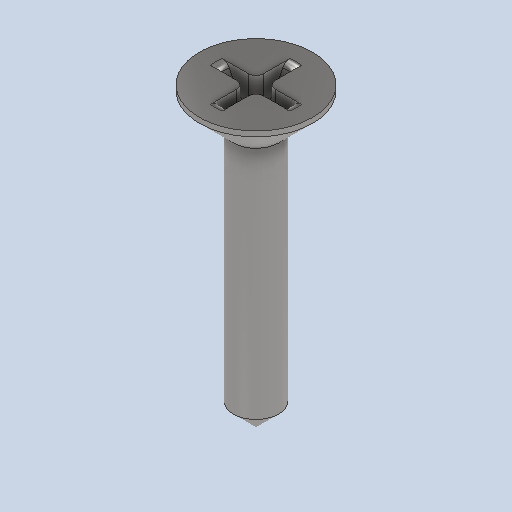
# Autodesk Inventor part: screw EE
Saved by Autodesk Inventor 2022 (Build 260153000, 153)
## iProperties
Created: 2021-06-28
Part Number: screw EE
Material: Iron, Malleable
Document SubType Name: Modeling
Designer: HP
Density: 7.15 g/cm^3
Appearance: Semi-Polished
Author: HP
Autodesk Inventor part; units mm, degrees
ref_plane "YZ Plane" through (0, 0, 0) normal (1, 0, 0) x (0, 1, 0)
ref_plane "XZ Plane" through (0, 0, 0) normal (0, 1, 0) x (-1, 0, 0)
ref_plane "XY Plane" through (0, 0, 0) normal (0, 0, 1) x (1, 0, 0)
sketch "Sketch1" plane through (0, 0, 0) normal (0, 0, 1) x (1, 0, 0)
  line L0 (0, -2.5) -> (0, -19)
  line L1 (0, -19) -> (1.4515, -17.5485)
  line L2 (1.4515, -17.5485) -> (1.4515, -2.5)
  line L3 (1.4515, -2.5) -> (3.625, -0.3265)
  line L4 (3.625, -0.3265) -> (3.625, 0)
  line L5 (3.625, 0) -> (2.25, 0)
  line L6 (0.7598, -2.0613) -> (0, -2.5)
  line L7 (0.7598, -2.0613) -> (1.5664, -1.466)
  line L8 (1.5664, -1.466) -> (2.25, 0)
  point P0 (0, 0)
  dimension "d0" = 3.625
  dimension "d1" = 2.25
  dimension "d2" = 19
  dimension "d3" = 60
  dimension "d4" = 45
  dimension "d5" = 2.5
  dimension "d6" = 2.5
  dimension "d7" = 25
  constraints: 18 end point, 3 parallel, 2 point on line, 1 perpendicular, 1 vertical
  measures "d0" distance from line of L0 L4.end
  measures "d1" distance from line of L0 L5.end
  measures "d2" distance from line of L0.end L5
  measures "d3" angle of L0 L6
  measures "d4" angle of L0 L3
  measures "d5" distance from line of L0.start L5
  measures "d6" distance from line of L2.end L5
  measures "d7" angle of L0 L8
revolve "Revolution1" add sketch "Sketch1" angle 360 about axis through (0, -2.5, 0) along (0, -1, 0)
sketch "Sketch2" plane through (0, 0, 0) normal (0, 1, 0) x (1, 0, 0)
  circle A0 centre (0, 0) radius 2.25 projected
  line L0 (0, 2.25) -> (0.375, 2.25)
  line L1 (0.375, 2.25) -> (-0.375, 2.25)
  line L2 (-0.375, 2.25) -> (-0.375, 0.875)
  line L3 (-0.875, 0.375) -> (-2.25, 0.375)
  line L4 (-2.25, 0.375) -> (-2.25, -0.375)
  line L5 (-2.25, -0.375) -> (-0.875, -0.375)
  line L6 (-0.375, -0.875) -> (-0.375, -2.25)
  line L7 (-0.375, -2.25) -> (0.375, -2.25)
  line L8 (0.375, -2.25) -> (0.375, -0.875)
  line L9 (0.875, -0.375) -> (2.25, -0.375)
  line L10 (2.25, -0.375) -> (2.25, 0.375)
  line L11 (2.25, 0.375) -> (0.875, 0.375)
  line L12 (0.375, 2.25) -> (0.375, 0.875)
  arc A1 (0.375, 0.875) -> (0.875, 0.375) centre (0.875, 0.875) ccw
  arc A2 (0.875, -0.375) -> (0.375, -0.875) centre (0.875, -0.875) ccw
  arc A3 (-0.375, -0.875) -> (-0.875, -0.375) centre (-0.875, -0.875) ccw
  arc A4 (-0.875, 0.375) -> (-0.375, 0.875) centre (-0.875, 0.875) ccw
  point P0 (0, 0)
  point P1 (-0.375, 0.375)
  point P2 (-0.375, -0.375)
  point P3 (0.375, -0.375)
  point P4 (0.375, 0.375)
  point P5 (-2.2185, -0.375)
  point P6 (-0.375, -2.2185)
  point P7 (0.375, -2.2185)
  point P8 (2.2185, -0.375)
  point P9 (2.2185, 0.375)
  point P10 (0.375, 2.2185)
  point P11 (-0.375, 2.2185)
  point P12 (-2.2185, 0.375)
  dimension "d9" = 0.375
  dimension "d10" = 0.75
  dimension "d11" = 1.875
  dimension "d12" = 1.875
  dimension "d13" = 0.75
  dimension "d14" = 1.875
  dimension "d15" = 1.875
  dimension "d16" = 0.5
  constraints: 26 end point, 16 point on line, 8 point on circle, 8 tangent, 7 perpendicular, 4 centre point, 3 equal radius, 2 horizontal, 1 vertical, 2 other
  measures "d9" distance of L0.start L0.end
  measures "d10" distance of L0.end L1.end
  measures "d11" distance of L1.end point (-0.375, 0.375)
  measures "d12" distance of point (-0.375, 0.375) L3.end
  measures "d13" distance of L3.end L4.end
  measures "d14" distance of point (-0.375, -0.375) L6.end
  measures "d15" distance of point (0.375, -0.375) L9.end
  measures "d16" radius of A1
extrude "Extrusion1" add sketch "Sketch2" against normal up to next contours L11 A1 L12 A0 | A0 L8 A2 L9 | L2 A4 L3 A0 | A0 L5 A3 L6
fillet "Fillet1" radius 0.5 4 edges at (-2.25, 0, 0) (0, 0, 2.25) (2.25, 0, 0) (0, 0, -2.25)
body "Solid1"
